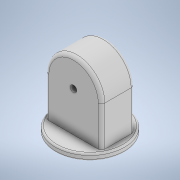
# Autodesk Inventor part: Base2
Saved by Autodesk Inventor 2021 (Build 250183000, 183)
## iProperties
Created: 2024-09-30
Part Number: Base2
Material: Generic
Document SubType Name: Modeling
Designer: Swoby
Density: 1 g/cm^3
Appearance: Default
Author: Swoby
Autodesk Inventor part; units mm, degrees
ref_plane "YZ Plane" through (0, 0, 0) normal (1, 0, 0) x (0, 1, 0)
ref_plane "XZ Plane" through (0, 0, 0) normal (0, 1, 0) x (-1, 0, 0)
ref_plane "XY Plane" through (0, 0, 0) normal (0, 0, 1) x (1, 0, 0)
sketch "Sketch1" plane through (0, 0, 0) normal (0, 0, 1) x (1, 0, 0)
  line L0 (0, 0) -> (50, 0)
  line L1 (52.5, 2.5) -> (52.5, 7.5)
  line L2 (50, 10) -> (0, 10)
  line L3 (0, 10) -> (0, 0)
  arc A0 (52.5, 7.5) -> (50, 10) centre (50, 7.5) ccw
  arc A1 (50, 0) -> (52.5, 2.5) centre (50, 2.5) ccw
  point P0 (52.5, 0)
  point P1 (52.5, 10)
  dimension "d0" = 105
  dimension "d1" = 10
  dimension "d2" = 2.5
  constraints: 8 end point, 4 point on circle, 4 point on line, 4 tangent, 3 perpendicular, 2 centre point, 1 equal radius, 1 horizontal
  measures "d0" diameter of L1 L3
  measures "d1" distance of point (52.5, 0) point (52.5, 10)
  measures "d2" radius of A0
revolve "Revolution1" add sketch "Sketch1" angle 360 about axis through (0, 10, 0) along (0, -1, 0)
sketch "Sketch2" plane through (0, 0, 0) normal (0, 0, 1) x (1, 0, 0)
  line L0 (-52.5, 2.5) -> (52.5, 2.5) projected
  line L1 (-50, 0) -> (50, 0) projected
  line L2 (-50, 10) -> (50, 10) projected
  line L3 (-52.5, 7.5) -> (52.5, 7.5) projected
  line L4 (-52.5, 7.5) -> (52.5, 7.5) projected
  line L5 (-52.5, 2.5) -> (52.5, 2.5) projected
  line L6 (-42.5, 10) -> (42.5, 10)
  line L7 (42.5, 10) -> (42.5, 70.7)
  line L8 (42.5, 70.7) -> (-42.5, 70.7) construction
  line L9 (-42.5, 70.7) -> (-42.5, 10)
  line L10 (0, 70.7) -> (0, 10) construction
  line L11 (-50, 10) -> (50, 10) projected
  arc A0 (42.5, 70.7) -> (-42.5, 70.7) centre (0, 70.7) ccw
  circle A1 centre (0, 70.7) radius 5
  point P0 (0, 0)
  point P1 (0, 0)
  dimension "d4" = 85
  dimension "d5" = 70.7
  dimension "d9" = 10
  constraints: 10 end point, 3 midpoint, 2 centre point, 2 parallel, 2 perpendicular, 2 point on circle, 2 point on line, 1 coincident, 1 horizontal, 1 tangent
  measures "d4" distance of L7.end L8.end
  measures "d5" distance of point (0, 0) L10.start
  measures "d9" diameter of A1
extrude "Extrusion1" add sketch "Sketch2" along normal mid plane 50
fillet "Fillet1" radius 5 6 edges at (-42.5, 40.35, 25) (42.5, 40.35, 25) (0, 113.2, 25) (42.5, 40.35, -25) (-42.5, 40.35, -25) (0, 113.2, -25)
body "Solid1"
